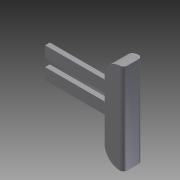
# Autodesk Inventor part: ThreadBreak
Saved by Autodesk Inventor 2012 SP2 (Build 160219200, 219)
## iProperties
Created: 2013-07-20
Part Number: ThreadBreak
Material: Default
Document SubType Name: Modeling
Designer: 1
Density: 1 g/cm^3
Author: 1
Autodesk Inventor part; units mm, degrees
ref_plane "YZ Plane" through (0, 0, 0) normal (1, 0, 0) x (0, 1, 0)
ref_plane "XZ Plane" through (0, 0, 0) normal (0, 1, 0) x (-1, 0, 0)
ref_plane "XY Plane" through (0, 0, 0) normal (0, 0, 1) x (1, 0, 0)
sketch "Sketch1" plane through (0, 0, 0) normal (0, 0, 1) x (1, 0, 0)
  line L0 (118.7984, -15.7076) -> (118.7984, -63.6601)
  line L1 (118.7984, -63.6601) -> (108.7984, -63.6601)
  line L2 (108.7984, -63.6601) -> (108.7984, -15.7076)
  line L3 (108.7984, -15.7076) -> (118.7984, -15.7076)
  line L4 (114.7984, 76.5) -> (114.7984, -850)
  point P0 (0, 0)
  dimension "d0" = 6
  dimension "d1" = 10
  constraints: 10 end point, 2 parallel, 2 vertical, 1 perpendicular, 2 other
  measures "d0" distance between parallel lines of L4 L2
  measures "d1" distance of L0.end L1.end
extrude "Extrusion1" add sketch "Sketch1" along normal mid plane 10
fillet "Fillet1" radius 8.35 2 edges at (108.7984, -15.7076, 0) (108.7984, -63.6601, 0)
fillet "Fillet2" radius 2 2 edges at (118.7984, -39.6839, -5) (118.7984, -39.6839, 5)
sketch "Sketch2" plane through (108.7984, -55.3101, 5) normal (-1, 0, 0) x (0, 0, 1)
  line L0 (-10, 31.2524) -> (0, 31.2524) projected
  line L1 (-6, 25.2524) -> (-4, 25.2524)
  line L2 (-4, 25.2524) -> (-4, 19.2524)
  line L3 (-4, 19.2524) -> (-6, 19.2524)
  line L4 (-6, 19.2524) -> (-6, 25.2524)
  line L5 (-5, 424.5751) -> (-5, -1099.7802)
  line L6 (-6, 15.2524) -> (-4, 15.2524)
  line L7 (-4, 15.2524) -> (-4, 9.2524)
  line L8 (-4, 9.2524) -> (-6, 9.2524)
  line L9 (-6, 9.2524) -> (-6, 15.2524)
  line L10 (-6.5, 55.3101) -> (-3.5, 55.3101) projected
  line L11 (-3.5, -794.6899) -> (-3.5, 55.3101) projected
  line L12 (-6.5, -794.6899) -> (-3.5, -794.6899) projected
  line L13 (-6.5, -794.6899) -> (-6.5, 55.3101) projected
  point P0 (-5, 55.3101)
  dimension "d6" = 1
  dimension "d7" = 2
  dimension "d8" = 6
  dimension "d9" = 6
  dimension "d12" = 10
  constraints: 18 end point, 2 parallel, 2 vertical, 1 collinear, 1 horizontal, 1 perpendicular, 9 other
  measures "d6" distance between parallel lines of L4 L5
  measures "d7" distance of L1.start L1.end
  measures "d8" distance of L1.end L2.end
  measures "d9" distance between parallel lines of L0 L1
  measures "d12" distance of L2.end L8.start
extrude "Extrusion2" add sketch "Sketch2" along normal blind 35.4 contours L5 L3 L4 L1 | L1 L2 L3 L5 | L8 L9 L6 L5 | L5 L6 L7 L8
sketch "Sketch3" plane through (0, 0, 5) normal (0, 0, 1) x (1, 0, 0)
  line L0 (108.7984, -55.3101) -> (108.7984, -24.0576) projected
  circle A0 centre (114.2984, -37.715) radius 3
  point P0 (116.7984, -15.715)
  point P1 (0, 0)
  dimension "d19" = 5.5
  dimension "d20" = 22
  dimension "d23" = 6
  constraints: 1 centre point
  measures "d19" distance from line of A0.centre L0
  measures "d20" vertical distance of A0.centre point (116.798, -15.715)
  measures "d23" diameter of A0
extrude "Extrusion3" add sketch "Sketch3" along normal mid plane 5
body "Solid1"
